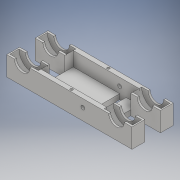
# Autodesk Inventor part: Водило
Saved by Autodesk Inventor 2017 (Build 210142000, 142)
## iProperties
Part Number: Водило
Material: Типовые
Document SubType Name: Modeling
Designer: Daemon
Density: 1 g/cm^3
Appearance: По умолчанию
Author: Daemon
Autodesk Inventor part; units mm, degrees
sketch "Эскиз1" plane through (0, 0, 0) normal (0, 0, 1) x (1, 0, 0)
  circle A0 centre (0, 0) radius 4
  circle A1 centre (0, 0) radius 11
  line L0 (-11, 0) -> (-12, 0)
  line L1 (-12, 0) -> (-12, -15)
  circle A2 centre (73, 0) radius 4
  circle A3 centre (73, 0) radius 11
  line L2 (84, 0) -> (85, 0)
  line L3 (85, 0) -> (85, -15)
  line L4 (-12, -15) -> (85, -15)
  line L5 (11, 0) -> (62, 0)
  dimension "d0" = 8
  dimension "d1" = 22
  dimension "d2" = 1
  dimension "d6" = 15
  dimension "d92" = 73
  dimension "d93" = 51
  constraints: 12 end point, 4 centre point, 4 horizontal, 4 point on circle, 3 coincident, 2 equal length, 2 equal radius, 2 vertical
  measures "d0" diameter of A0
  measures "d1" diameter of A1
  measures "d2" distance of L0.start L0.end
  measures "d6" distance of L0.end L1.end
  measures "d92" distance of point (0, 0) A2.centre
  measures "d93" distance of L5.start L5.end
extrude "Выдавливание1" add sketch "Эскиз1" along normal blind 32 contours L5 A3 L2 L3 L4 L1 L0 A1
sketch "Эскиз2" plane through (0, 0, 32) normal (0, 0, 1) x (1, 0, 0)
  arc A0 (-11, 0) -> (11, 0) centre (0, 0) ccw
  line L0 (62, 0) -> (11, 0) projected
  arc A1 (-11, 0) -> (11, 0) centre (0, 0) ccw projected
  line L1 (11, 0) -> (11, 0)
  arc A2 (-6, 0) -> (6, 0) centre (0, 0) ccw
  line L2 (-11, 0) -> (-6, 0)
  line L3 (6, 0) -> (11, 0)
  dimension "d14" = 12
  constraints: 6 end point, 4 point on circle, 3 horizontal, 2 centre point, 2 coincident
  measures "d14" diameter of A2
extrude "Выдавливание2" add sketch "Эскиз2" against normal blind 1.5
sketch "Эскиз3" plane through (0, 0, 32) normal (0, 0, 1) x (1, 0, 0)
  arc A0 (62, 0) -> (84, 0) centre (73, 0) ccw projected
  line L0 (85, 0) -> (84, 0) projected
  line L1 (84, 0) -> (84, 0)
  arc A1 (62, 0) -> (84, 0) centre (73, 0) ccw
  arc A2 (67.0053, 0) -> (78.9947, 0) centre (73, 0) ccw
  line L2 (62, 0) -> (11, 0) projected
  line L3 (62, 0) -> (67.0053, 0)
  line L4 (78.9947, 0) -> (84, 0)
  point P0 (0, 0)
  constraints: 6 end point, 4 point on circle, 2 centre point, 2 coincident, 2 horizontal, 1 collinear
extrude "Выдавливание3" add sketch "Эскиз3" against normal blind 1.5
ref_plane "РабПлоскость5" through (0, 0, 16) normal (0, 0, -1) x (-1, 0, 0)
mirror "Зеркальное отражение7" about plane through (0, 0, 16) normal (0, 0, -1) of "Выдавливание3"
mirror "Зеркальное отражение8" about plane through (0, 0, 16) normal (0, 0, -1) of "Выдавливание2"
ref_plane "РабПлоскость10" through (0, 0, 27) normal (0, 0, 1) x (1, 0, 0)
mirror "Зеркальное отражение9" about plane through (0, 0, 27) normal (0, 0, 1) of "Выдавливание2"
mirror "Зеркальное отражение10" about plane through (0, 0, 27) normal (0, 0, 1) of "Выдавливание3"
ref_plane "РабПлоскость11" through (0, 0, 5) normal (0, 0, -1) x (-1, 0, 0)
mirror "Зеркальное отражение11" about plane through (0, 0, 5) normal (0, 0, -1) of "Зеркальное отражение8"
mirror "Зеркальное отражение12" about plane through (0, 0, 5) normal (0, 0, -1) of "Зеркальное отражение7"
sketch "Эскиз14" plane through (6, 0, 30.5) normal (0, 1, 0) x (1, 0, 0)
  line L0 (5, 20.5) -> (5, 8.5) projected
  line L1 (5, 14.5) -> (56, 14.5)
  line L2 (56, 20.5) -> (56, 8.5) projected
  line L3 (56, 14.5) -> (56, 27)
  line L4 (56, 29) -> (56, 22) projected
  line L5 (5, 14.5) -> (5, 27)
  line L6 (5, 29) -> (5, 22) projected
  line L7 (5, 27) -> (56, 27)
  dimension "d94" = 12.5
  constraints: 8 end point, 2 midpoint, 2 point on line, 1 perpendicular
  measures "d94" distance of L1.end L3.end
extrude "Выдавливание11" cut sketch "Эскиз14" against normal blind 11
ref_plane "РабПлоскость14" through (36.5, -15, 0) normal (-1, 0, 0) x (0, 0, 1)
sketch "Эскиз15" plane through (85, 0, 32) normal (0, 1, 0) x (1, 0, 0)
  line L0 (-23, 16) -> (-23, 10) projected
  line L1 (-23, 10) -> (9, 10)
  line L2 (9, 10) -> (9, 22)
  line L3 (9, 22) -> (-23, 22)
  line L4 (-23, 22) -> (-23, 10)
  point P0 (-85, 32)
  dimension "d95" = 12
  dimension "d96" = 32
  constraints: 8 end point, 2 parallel, 1 horizontal, 1 perpendicular
  measures "d95" distance of L1.end L2.end
  measures "d96" distance of L0.end L1.end
extrude "Выдавливание12" cut sketch "Эскиз15" against normal up to next
mirror "Зеркальное отражение15" about plane through (36.5, -15, 0) normal (-1, 0, 0) of "Выдавливание12"
sketch "Эскиз16" plane through (6, 0, 30.5) normal (0, 1, 0) x (1, 0, 0)
  line L0 (79, 8.5) -> (79, -1.5) projected
  line L1 (-18, 30.5) -> (-18, -1.5) projected
  line L2 (61.0053, -1.5) -> (0, -1.5) projected
  line L3 (30.5026, -1.5) -> (30.5026, 0.25)
  circle A0 centre (30.5026, 0.25) radius 1
  point P0 (-6, 30.5)
  point P1 (-18, 8.5)
  dimension "d86" = 1.75
  dimension "d87" = 2
  constraints: 2 end point, 1 centre point, 1 coincident, 1 midpoint, 1 vertical
  measures "d86" distance of L3.start L3.end
  measures "d87" diameter of A0
extrude "Выдавливание13" cut sketch "Эскиз16" against normal up to next
mirror "Зеркальное отражение16" about plane through (0, 0, 16) normal (0, 0, -1) of "Выдавливание13"
mirror "Зеркальное отражение17" about plane through (0, 0, 16) normal (0, 0, -1) of "Выдавливание11"
sketch "Эскиз19" plane through (62, 0, 28.5) normal (0, 0, -1) x (-1, 0, 0)
  circle A0 centre (36, -6) radius 1.5
  line L0 (51, -11) -> (0, -11) projected
  line L1 (51, 0) -> (51, -11) projected
  point P0 (62, 0)
  dimension "d103" = 3
  dimension "d104" = 5
  dimension "d105" = 15
  constraints: 1 centre point
  measures "d103" diameter of A0
  measures "d104" distance from line of L0 A0.centre
  measures "d105" distance from line of L1 A0.centre
extrude "Выдавливание15" cut sketch "Эскиз19" against normal up to next
mirror "Зеркальное отражение18" about plane through (0, 0, 16) normal (0, 0, -1) of "Выдавливание15"
sketch "Эскиз20" plane through (6, -11, 30.5) normal (0, 1, 0) x (1, 0, 0)
  line L0 (5, 27) -> (56, 27) projected
  line L1 (5, 2) -> (56, 2) projected
  line L2 (5, 8.5) -> (5, 20.5) projected
  line L3 (5, 27) -> (56, 27) projected
  line L4 (56, 2) -> (5, 2) projected
  line L5 (15, 27) -> (20, 27)
  line L6 (20, 27) -> (20, 2)
  line L7 (20, 2) -> (15, 2)
  line L8 (15, 2) -> (15, 27)
  point P0 (-6, 30.5)
  dimension "d119" = 5
  dimension "d120" = 15
  constraints: 8 end point, 2 parallel, 2 point on line, 1 horizontal, 1 perpendicular
  measures "d119" distance between parallel lines of L8 L6
  measures "d120" distance between parallel lines of L2 L6
extrude "Выдавливание17" cut sketch "Эскиз20" against normal up to next
